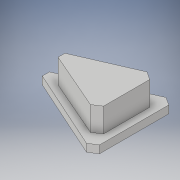
# Autodesk Inventor part: SideButton
Saved by Autodesk Inventor 2019 (Build 230136000, 136)
## iProperties
Created: 2021-04-22
Part Number: SideButton
Material: Všeobecné
Document SubType Name: Modeling
Designer: miko flosso
Density: 1 g/cm^3
Appearance: Výchozí
Author: miko flosso
Autodesk Inventor part; units mm, degrees
ref_plane "YZ Plane" through (0, 0, 0) normal (1, 0, 0) x (0, 1, 0)
ref_plane "XZ Plane" through (0, 0, 0) normal (0, 1, 0) x (-1, 0, 0)
ref_plane "XY Plane" through (0, 0, 0) normal (0, 0, 1) x (1, 0, 0)
sketch "Náčrt1" plane through (0, 0, 0) normal (0, 1, 0) x (-1, 0, 0)
  line L0 (-10, 0) -> (-10, -9)
  line L1 (-10, -9) -> (0, -4.5)
  line L2 (-10, 0) -> (0, -4.5)
  point P0 (0, 0)
  dimension "d1" = 9
  constraints: 6 end point
  measures "d1" distance of L0.end L0.start
extrude "Vysunutí1" add sketch "Náčrt1" along normal blind 0.8
sketch "Náčrt2" plane through (0, 0.8, 0) normal (0, 1, 0) x (1, 0, 0)
  line L0 (9.22, 1.2) -> (9.22, 7.8)
  line L1 (10, 0) -> (10, 9) projected
  line L2 (9.22, 7.8) -> (1.62, 4.5)
  line L3 (9.22, 1.2) -> (1.62, 4.5)
  point P0 (0, 0)
  dimension "d6" = 0.78
  constraints: 6 end point
  measures "d6" distance between parallel lines of L0 L1
extrude "Vysunutí2" add sketch "Náčrt2" along normal blind 2.5
chamfer "Zkosení1" distance 0.9 angle 45 3 edges at (1.62, 2.05, -4.5) (9.22, 2.05, -1.2) (9.22, 2.05, -7.8)
chamfer "Zkosení2" distance 0.9 angle 45 3 edges at (10, 0.4, 0) (10, 0.4, -9) (0, 0.4, -4.5)
